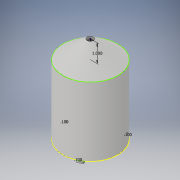
# Autodesk Inventor part: engine_mount_MkI
Saved by Autodesk Inventor 2017 (Build 210142000, 142)
## iProperties
Created: 2017-11-28
Part Number: engine_mount_MkI
Material: Generic
Document SubType Name: Modeling
Designer: Harrison
Density: 1 g/cm^3
Appearance: Default
Author: Harrison
Autodesk Inventor part; units mm, degrees
ref_plane "YZ Plane" through (0, 0, 0) normal (1, 0, 0) x (0, 1, 0)
ref_plane "XZ Plane" through (0, 0, 0) normal (0, 1, 0) x (-1, 0, 0)
ref_plane "XY Plane" through (0, 0, 0) normal (0, 0, 1) x (1, 0, 0)
sketch "Sketch1" plane through (0, 0, 0) normal (0, 1, 0) x (-1, 0, 0)
  circle A0 centre (0, 0) radius 12.192
  circle A1 centre (0, -37.084) radius 12.192
  line L0 (0, 0) -> (37.084, 0) construction
  circle A2 centre (-32.1157, -18.542) radius 12.192
  line L1 (0, 0) -> (49.1792, 0) construction
  circle A3 centre (-10.7052, -18.542) radius 38.608
  dimension "d0" = 24.384
  dimension "d6" = 24.384
  dimension "d10" = 24.384
  constraints: 4 centre point, 4 end point, 2 horizontal, 1 coincident
  measures "d0" diameter of A0
  measures "d6" diameter of A1
  measures "d10" diameter of A2
extrude "Extrusion1" add sketch "Sketch1" along normal blind 96.52
sketch "Sketch2" plane through (10.7052, 96.52, -18.542) normal (0, 1, 0) x (1, 0, 0)
  circle A0 centre (0, 0) radius 38.608
  point P0 (-10.7052, -18.542)
  constraints: 1 centre point
sketch3d "3D Sketch1"
ref_plane "Work Plane3" through (10.7052, 96.52, -18.542) normal (-0.4271799, 0, 0.9041667) x (0, -1, 0)
sketch "Sketch4" plane through (10.7052, 96.52, -18.542) normal (-0.4271799, 0, 0.9041667) x (0, -1, 0)
  line L0 (-25.4, 0) -> (-25.4, 4.445)
  line L1 (0, 38.608) -> (0, -38.608) projected
  line L2 (-25.4, 4.445) -> (0, 38.608)
  line L3 (0, 26.3793) -> (-21.4115, 4.445)
  line L4 (-21.4115, 4.445) -> (-25.4, 4.445)
  line L5 (0, 0) -> (-25.4, 0)
  point P0 (96.52, -1.7585)
  dimension "d17" = 4.445
  constraints: 10 end point, 2 horizontal, 1 midpoint, 1 point on line, 1 vertical
  measures "d17" distance of L0.start L0.end
revolve "Revolution1" add sketch "Sketch4" angle 360 about axis through (10.7052, 96.52, -18.542) along (0, 1, 0) contours L2 L1 L3 L4
sketch "Sketch5" plane through (10.7052, 0, -18.542) normal (0, -1, 0) x (1, 0, 0)
  circle A0 centre (0, 0) radius 38.608 projected
  line L0 (-38.608, 0) -> (-34.798, 0) construction
  line L1 (-38.4195, -3.81) -> (-35.8662, -3.81)
  line L2 (-38.608, 0) -> (-34.798, 0) construction
  line L3 (-38.4195, 3.81) -> (-35.8662, 3.81)
  line L4 (-35.8662, 3.81) -> (-35.8651, 3.81)
  line L5 (-35.8662, -3.81) -> (-35.8639, -3.81)
  line L6 (14.6335, 32.966) -> (15.9102, 35.1773)
  line L7 (21.2327, 29.156) -> (22.5093, 31.3673)
  line L8 (21.2327, -29.156) -> (22.5093, -31.3673)
  line L9 (14.6335, -32.966) -> (15.9102, -35.1773)
  arc A1 (21.2327, 29.156) -> (14.6335, 32.966) centre (0, 0) ccw
  arc A2 (21.7434, 30.0407) -> (15.1443, 33.8507) centre (0, 0) ccw
  arc A3 (-35.8662, 3.81) -> (-35.8662, -3.81) centre (0, 0) ccw
  arc A4 (14.6335, -32.966) -> (21.2327, -29.156) centre (0, 0) ccw
  arc A5 (-36.8878, 3.81) -> (-36.8878, -3.81) centre (0, 0) ccw
  arc A6 (15.1443, -33.8507) -> (21.7434, -30.0407) centre (0, 0) ccw
  arc A7 (-38.4195, 3.81) -> (-38.4195, -3.81) centre (0, 0) ccw
  arc A8 (15.9102, -35.1773) -> (22.5093, -31.3673) centre (0, 0) ccw
  arc A9 (22.5093, 31.3673) -> (15.9102, 35.1773) centre (0, 0) ccw
  line L10 (22.5093, -31.3673) -> (20.3981, -32.7795)
  line L11 (20.3981, -32.7795) -> (19.1274, -30.5785)
  line L12 (-38.4195, -3.81) -> (-38.5869, -1.2755)
  line L13 (15.9102, 35.1773) -> (18.1888, 34.055)
  line L14 (18.1888, 34.055) -> (16.9181, 31.854)
  line L15 (-38.5869, -1.2755) -> (-36.0454, -1.2755)
  point P0 (-10.7052, 18.542)
  dimension "d33" = 2.54
  dimension "d34" = 2.54
  dimension "d35" = 2.54
  constraints: 32 end point, 27 point on circle, 9 centre point, 6 horizontal, 6 point on line, 2 coincident
  measures "d33" distance of L8.end L10.end
  measures "d34" distance of L1.start L12.end
  measures "d35" distance of L6.end L13.end
extrude "Extrusion2" add sketch "Sketch5" along normal blind 3.175 contours L7 A2 L14 A0 | L10 L11 A6 L8 | A0 L10 | L13 A0 | L14 A2 L6 L13 | A0 L9 A6 L11 | L3 A5 L15 A0 | L12 L15 A5 L1 | A0 L12
extrude "Extrusion3" add sketch "Sketch5" along normal blind 3.175 contours L7 A2 L14 A0 | L10 L11 A6 L8 | L7 A1 L14 A2 | A0 L9 A6 L11 | A6 L9 A4 L11 | L3 A5 L15 A0 | L3 A3 L15 A5
extrude "Extrusion4" add sketch "Sketch5" along normal blind 3.175 separate body contours L7 A1 L14 A2 | A6 L11 A4 L8 | L14 A1 L6 A2 | A6 L9 A4 L11 | L3 A3 L15 A5 | A5 L15 A3 L1
extrude "Extrusion5" cut sketch "Sketch5" along normal blind 1.5875 contours L3 A3 L15 A5 | A5 L15 A3 L1 bodies 1
extrude "Extrusion6" cut sketch "Sketch5" along normal blind 1.5875 contours L3 A3 L15 A5 | A5 L15 A3 L1 bodies 1
extrude "Extrusion7" add sketch "Sketch5" along normal blind 1.5875 contours L3 A3 L15 A5 | A5 L15 A3 L1 bodies 1
extrude "Extrusion8" cut sketch "Sketch5" along normal blind 1.5875 contours L3 A5 L15 A0 | L3 A3 L15 A5 bodies 1 2
extrude "Extrusion9" cut sketch "Sketch5" along normal blind 1.5875 contours L7 A2 L14 A0 | L7 A1 L14 A2 bodies 1 2
extrude "Extrusion10" cut sketch "Sketch5" along normal blind 1.5875 contours A0 L9 A6 L11 | A6 L9 A4 L11 bodies 1
extrude "Extrusion11" cut sketch "Sketch5" along normal blind 1.5875 contours A0 L9 A6 L11 | A6 L9 A4 L11 bodies 1 2
body "Solid1"
body "Solid2"
